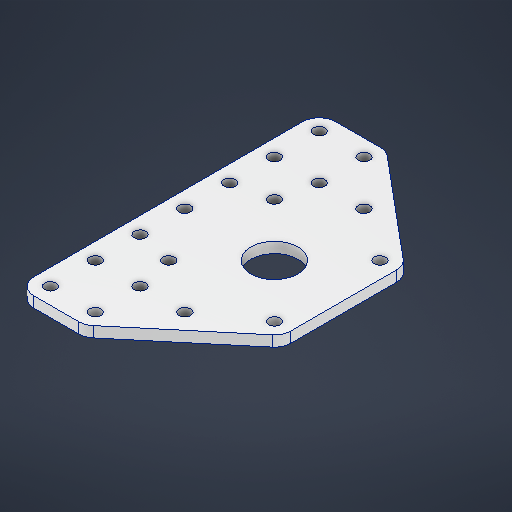
# Autodesk Inventor part: CNC-008-XAxisNema23Mount
Saved by Autodesk Inventor 2026.2 (Build 302298000, 298)
## iProperties
Created: 2026-06-15
Part Number: CNC-008-XAxisNema23Mount
Material: Aluminum 6061
Document SubType Name: Modeling
Designer: Kenji
Density: 2.7 g/cm^3
Appearance: Aluminum - Flat
Author: Kenji
Autodesk Inventor part; units mm, degrees
ref_plane "YZ Plane" through (0, 0, 0) normal (1, 0, 0) x (0, 1, 0)
ref_plane "XZ Plane" through (0, 0, 0) normal (0, 1, 0) x (-1, 0, 0)
ref_plane "XY Plane" through (0, 0, 0) normal (0, 0, 1) x (1, 0, 0)
sketch "Sketch1" plane through (0, 0, 0) normal (0, 1, 0) x (-1, 0, 0)
  circle A0 centre (0, 0) radius 2.6
  line L0 (0, 0) -> (0, -2.6) construction
  line L1 (0, 0) -> (-2.6, 0) construction
  circle A1 centre (0, -20) radius 2.6
  circle A2 centre (0, -40) radius 2.6
  circle A3 centre (0, -60) radius 2.6
  circle A4 centre (0, -80) radius 2.6
  circle A5 centre (0, -100) radius 2.6
  circle A6 centre (0, -120) radius 2.6
  circle A7 centre (-20, 0) radius 2.6
  circle A8 centre (-20, -120) radius 2.6
  circle A9 centre (-40, -60) radius 10.5
  circle A10 centre (-16.43, -36.43) radius 2.6
  circle A11 centre (-16.43, -83.57) radius 2.6
  circle A12 centre (-63.57, -83.57) radius 2.6
  circle A13 centre (-63.57, -36.43) radius 2.6
  circle A14 centre (-20, -100) radius 2.6
  circle A15 centre (-40, -100) radius 2.6
  circle A16 centre (-20, -20) radius 2.6
  circle A17 centre (-40, -20) radius 2.6
  circle A18 centre (0, 0) radius 7.3625 construction
  circle A19 centre (-20, 0) radius 7.3625 construction
  circle A20 centre (-40, -20) radius 7.3625 construction
  circle A21 centre (-63.57, -36.43) radius 7.3625 construction
  circle A22 centre (-63.57, -83.57) radius 7.3625 construction
  circle A23 centre (-40, -100) radius 7.3625 construction
  circle A24 centre (-20, -120) radius 7.3625 construction
  circle A25 centre (0, -120) radius 7.3625 construction
  line L2 (7.3625, 0) -> (7.3625, -120)
  line L3 (0, -127.3625) -> (-20, -127.3625)
  line L4 (0, 7.3625) -> (-20, 7.3625)
  line L5 (-24.7227, 5.6483) -> (-68.2927, -30.7817)
  line L6 (-70.9325, -36.43) -> (-70.9325, -83.57)
  line L7 (-68.2927, -89.2183) -> (-24.7227, -125.6483)
  arc A26 (0, -127.3625) -> (7.3625, -120) centre (0, -120) ccw
  arc A27 (-24.7227, -125.6483) -> (-20, -127.3625) centre (-20, -120) ccw
  arc A28 (-70.9325, -83.57) -> (-68.2927, -89.2183) centre (-63.57, -83.57) ccw
  arc A29 (-68.2927, -30.7817) -> (-70.9325, -36.43) centre (-63.57, -36.43) ccw
  arc A30 (-20, 7.3625) -> (-24.7227, 5.6483) centre (-20, 0) ccw
  arc A31 (7.3625, 0) -> (0, 7.3625) centre (0, 0) ccw
  point P0 (0, -22.6)
  point P1 (-2.6, -20)
  point P2 (0, -42.6)
  point P3 (-2.6, -40)
  point P4 (0, -62.6)
  point P5 (-2.6, -60)
  point P6 (0, -82.6)
  point P7 (-2.6, -80)
  point P8 (0, -102.6)
  point P9 (-2.6, -100)
  point P10 (0, -122.6)
  point P11 (-2.6, -120)
  dimension "d0" = 5.2
  dimension "d3" = 20
  dimension "d8" = 20
  dimension "d9" = 40
  dimension "d10" = 60
  dimension "d11" = 21
  dimension "d12" = 23.57
  dimension "d13" = 23.57
  dimension "d14" = 23.57
  dimension "d15" = 23.57
  dimension "d16" = 20
  dimension "d17" = 4.7625
  constraints: 38 point on circle, 32 centre point, 23 equal radius, 16 end point, 13 tangent, 8 coincident, 7 horizontal alignment, 6 vertical alignment, 2 horizontal, 2 vertical, 1 point on line, 24 other
  measures "d0" diameter of A0
  measures "d3" distance of L0.start A1.centre
  measures "d8" distance of A7.centre point (0, 0)
  measures "d9" horizontal distance of A9.centre point (0, 0)
  measures "d10" vertical distance of A9.centre point (0, 0)
  measures "d11" diameter of A9
  measures "d12" horizontal distance of A9.centre A10.centre
  measures "d13" horizontal distance of A9.centre A10.centre
  measures "d14" horizontal distance of A11.centre A9.centre
  measures "d15" horizontal distance of A13.centre A9.centre
  measures "d16" distance of A15.centre A14.centre
  measures "d17" radial gap between concentric circles of A18 A0
extrude "Extrusion1" add sketch "Sketch1" along normal blind 4.7625
equation "\"d14\" = d13"
equation "\"d15\" = d12"
body "Solid1"
